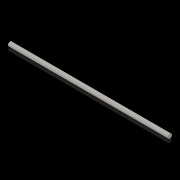
# Autodesk Inventor part: Shaft
Saved by Autodesk Inventor 2020 (Build 240168000, 168)
## iProperties
Created: 2020-08-27
Part Number: Shaft
Material: Steel
Document SubType Name: Modeling
Designer: alons
Density: 1 g/cm^3
Appearance: Steel
CustomPartVersion: 1
Author: alons
Length: 11.000 mm
Autodesk Inventor part; units mm, degrees
ref_plane "Start Plane" through (0, 0, 0) normal (1, 0, 0) x (0, 1, 0)
ref_plane "XZ Plane" through (0, 0, 0) normal (0, 1, 0) x (-1, 0, 0)
ref_plane "XY Plane" through (0, 0, 0) normal (0, 0, 1) x (1, 0, 0)
sketch "Main Sketch" plane through (0, 0, 0) normal (0, 0, 1) x (1, 0, 0)
  line L0 (0, 0) -> (11, 0)
  line L1 (0, 0) -> (0, 0.625)
  line L2 (0, 0.625) -> (0.5, 0.625)
  line L3 (0.5, 0.5) -> (7.5, 0.5)
  line L4 (7.5, 0.575) -> (8, 0.575)
  line L5 (8, 0.5) -> (11, 0.5)
  line L6 (11.7188, 0.25) -> (12.2188, 0.25)
  line L7 (12.2188, 0.25) -> (17.2188, 0.25)
  line L8 (19.2188, 0.25) -> (19.2188, 0)
  line L9 (17.2188, 0.25) -> (19.2188, 0.25)
  line L10 (0.5, 0.625) -> (0.5, 0.5)
  line L11 (11, 0.5) -> (11, 0)
  line L12 (7.5, 0.5) -> (7.5, 0.575)
  line L13 (8, 0.575) -> (8, 0.5)
  dimension "d3" = 1.25
  dimension "d4" = 1
  dimension "d5" = 1.15
  dimension "d6" = 1
  dimension "d7" = 0.5
  dimension "d8" = 0.5
  dimension "d9" = 0.5
  constraints: 28 end point, 6 vertical, 4 horizontal
  measures "d3" diameter of L2 L0
  measures "d4" diameter of L3 L0
  measures "d5" diameter of L4 L0
  measures "d6" diameter of L5 L0
  measures "d7" diameter of L6 L0
  measures "d8" diameter of L7 L0
  measures "d9" diameter of L9 L0
revolve "Revolution1" add sketch "Main Sketch" angle 360 about axis through (0, 0, 0) along (1, 0, 0)
equation "\"Length\" = 11"
body "Solid1"
